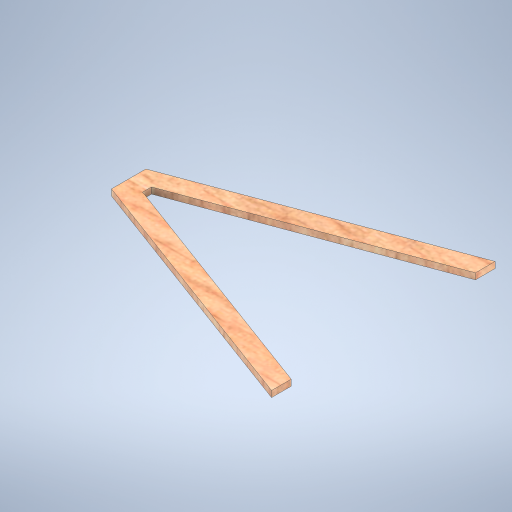
# Autodesk Inventor part: Projectile Launcher Back
Saved by Autodesk Inventor 2024 (Build 280153000, 153)
## iProperties
Created: 2023-09-26
Part Number: Projectile Launcher Back
Material: Wood (Birch)
Document SubType Name: Modeling
Designer: Nick
Density: 0.55 g/cm^3
Appearance: Birch - Natural Polished
Author: Nick
Autodesk Inventor part; units mm, degrees
ref_plane "YZ Plane" through (0, 0, 0) normal (1, 0, 0) x (0, 1, 0)
ref_plane "XZ Plane" through (0, 0, 0) normal (0, 1, 0) x (-1, 0, 0)
ref_plane "XY Plane" through (0, 0, 0) normal (0, 0, 1) x (1, 0, 0)
sketch "Sketch1" plane through (0, 0, 0) normal (0, 1, 0) x (-1, 0, 0)
  line L0 (0, 0) -> (0, -10.16)
  line L1 (0, -10.16) -> (166.6875, -72.0318)
  line L2 (166.6875, -72.0318) -> (170.0021, -63.1021)
  line L3 (170.0021, -63.1021) -> (0, 0)
  line L4 (0, -133.9036) -> (166.6875, -72.0318)
  line L5 (170.0021, -80.9615) -> (0, -144.0636)
  line L6 (0, -144.0636) -> (0, -133.9036)
  line L7 (166.6875, -72.0318) -> (170.0021, -80.9615)
  line L8 (170.0021, -63.1021) -> (160.4771, -63.1021)
  line L9 (160.4771, -63.1021) -> (160.4771, -80.9615)
  line L10 (160.4771, -80.9615) -> (170.0021, -80.9615)
  line L11 (170.0021, -80.9615) -> (170.0021, -63.1021)
  line L12 (0, 0) -> (38.1, 0)
  line L13 (38.1, 0) -> (38.1, -144.0636)
  line L14 (38.1, -144.0636) -> (0, -144.0636)
  line L15 (0, -144.0636) -> (0, 0)
  point P0 (160.4771, -69.7266)
  point P1 (160.4771, -74.337)
  dimension "d0" = 10.16
  dimension "d1" = 9.525
  dimension "d2" = 177.8
  dimension "d3" = 177.8
  dimension "d4" = 10.16
  dimension "d5" = 9.525
  dimension "d6" = 9.525
  dimension "d9" = 38.1
  constraints: 32 end point, 5 parallel, 5 perpendicular, 2 horizontal, 2 point on line, 1 collinear, 1 vertical
  measures "d0" distance of L0.start L0.end
  measures "d1" distance of L1.end L2.end
  measures "d2" distance of L0.end L1.end
  measures "d3" distance of L4.start L1.end
  measures "d4" distance of L5.end L4.start
  measures "d5" distance of L1.end L5.start
  measures "d6" distance of L10.end L9.end
  measures "d9" distance of L13.end L14.end
extrude "Extrusion1" add sketch "Sketch1" along normal blind 3.175 contours L3 L13 L1 L0 | L3 L8 L9 L1 L13 | L4 L13 L5 L6 | L11 L7 L2 | L2 L1 L9 L8 | L1 L4 L9 | L4 L9 L10 L5 L13 | L7 L10 L9 L4
sketch "Sketch2" plane through (0, 3.175, 0) normal (0, 1, 0) x (1, 0, 0)
  line L0 (0, 0) -> (0, 10.16) projected
  line L1 (0, 0) -> (-38.1, 0)
  line L2 (-38.1, 0) -> (-38.1, 144.0636)
  line L3 (-38.1, 144.0636) -> (0, 144.0636)
  line L4 (0, 144.0636) -> (0, 0)
  dimension "d10" = 38.1
  constraints: 8 end point, 2 parallel, 1 horizontal, 1 perpendicular
  measures "d10" distance of L2.end L3.end
extrude "Extrusion2" cut sketch "Sketch2" against normal blind 3.175
body "Solid1"
